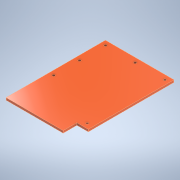
# Autodesk Inventor part: Gas Side Top Cover
Saved by Autodesk Inventor 2021 (Build 250183000, 183)
## iProperties
Created: 2020-08-17
Part Number: Gas Side Top Cover
Material: Generic
Document SubType Name: Modeling
Designer: jgray
Density: 1 g/cm^3
Appearance: Default
Author: jgray
Autodesk Inventor part; units mm, degrees
ref_plane "YZ Plane" through (0, 0, 0) normal (1, 0, 0) x (0, 1, 0)
ref_plane "XZ Plane" through (0, 0, 0) normal (0, 1, 0) x (-1, 0, 0)
ref_plane "XY Plane" through (0, 0, 0) normal (0, 0, 1) x (1, 0, 0)
sketch "Sketch1" plane through (0, 0, 0) normal (0, 1, 0) x (-1, 0, 0)
  line L0 (0, 0) -> (90, 0)
  line L1 (90, 0) -> (90, -112.5)
  line L2 (90, -112.5) -> (0, -112.5)
  line L3 (0, -112.5) -> (0, 0)
  dimension "d0" = 90
  dimension "d1" = 112.5
  constraints: 8 end point, 2 parallel, 1 horizontal, 1 perpendicular
  measures "d0" distance of L1.end L2.end
  measures "d1" distance of L0.end L1.end
extrude "Extrusion1" add sketch "Sketch1" along normal blind 3
sketch "Sketch3" plane through (-90, 0, 0) normal (0, 0, 1) x (1, 0, 0)
  line L0 (90, 0) -> (0, 0) projected
  line L1 (90, 3) -> (0, 3) projected
  line L2 (0, 0) -> (75, 0)
  line L3 (75, 0) -> (75, 3)
  line L4 (75, 3) -> (0, 3)
  line L5 (0, 3) -> (0, 0)
  line L6 (90, 0) -> (90, 3) projected
  point P0 (0, 3)
  dimension "d5" = 15
  constraints: 8 end point, 2 parallel, 1 horizontal, 1 perpendicular, 1 point on line
  measures "d5" distance between parallel lines of L6 L3
extrude "Extrusion2" add sketch "Sketch3" along normal blind 18 contours L0 L5 L1 L3
sketch "Sketch4" plane through (0, 3, 0) normal (0, 1, 0) x (1, 0, 0)
  line L0 (-6, 128.5084) -> (-6, -27.8518) construction
  line L1 (-118.0415, 106.5) -> (21.4799, 106.5) construction
  line L2 (-84, 125.301) -> (-84, -43.3542) construction
  line L3 (-90, 112.5) -> (-90, -18) projected
  line L4 (0, 112.5) -> (-90, 112.5) projected
  line L5 (0, 0) -> (0, 112.5) projected
  line L6 (-35.7185, 6) -> (24.9546, 6) construction
  line L7 (-15, 0) -> (0, 0) projected
  point P0 (-7.5, 6)
  point P1 (-6, 106.5)
  point P2 (-45, 106.5)
  point P3 (-84, 106.5)
  point P4 (-84, 72.5)
  point P5 (-84, 38.5)
  dimension "d8" = 6
  dimension "d9" = 6
  dimension "d10" = 6
  dimension "d11" = 6
  dimension "d12" = 7.5
  dimension "d13" = 39
  dimension "d14" = 34
  dimension "d15" = 34
  constraints: 8 end point, 8 point on line, 2 horizontal, 2 vertical
  measures "d8" distance between parallel lines of L3 L2
  measures "d9" distance between parallel lines of L1 L4
  measures "d10" distance between parallel lines of L5 L0
  measures "d11" distance between parallel lines of L7 L6
  measures "d12" distance from line of L5 point (-7.5, 6)
  measures "d13" distance of point (-84, 106.5) point (-45, 106.5)
  measures "d14" distance of point (-84, 72.5) point (-84, 106.5)
  measures "d15" distance of point (-84, 72.5) point (-84, 38.5)
hole "Hole1" at (-7.5, 3, -6) at (-6, 3, -106.5) at (-45, 3, -106.5) at (-84, 3, -106.5) at (-84, 3, -72.5) at (-84, 3, -38.5) direction (0, -1, 0) diameter 3.2 end through all
body "Solid1"
